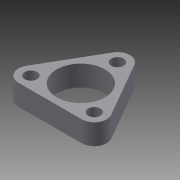
# Autodesk Inventor part: 零件3
Saved by Autodesk Inventor 2014 (Build 180170000, 170)
## iProperties
Created: 2018-10-26
Part Number: 零件3
Material: 常规
Document SubType Name: Modeling
Designer: Administrator
Density: 1 g/cm^3
Appearance: 默认
Author: Administrator
Autodesk Inventor part; units mm, degrees
ref_plane "YZ Plane" through (0, 0, 0) normal (1, 0, 0) x (0, 1, 0)
ref_plane "XZ Plane" through (0, 0, 0) normal (0, 1, 0) x (-1, 0, 0)
ref_plane "XY Plane" through (0, 0, 0) normal (0, 0, 1) x (1, 0, 0)
sketch "草图1" plane through (0, 0, 0) normal (0, 0, 1) x (1, 0, 0)
  line L0 (-7.7942, 31) -> (-30.7439, -8.75)
  line L1 (-22.9497, -22.25) -> (22.9497, -22.25)
  line L2 (7.7942, 31) -> (30.7439, -8.75)
  arc A0 (-30.7439, -8.75) -> (-22.9497, -22.25) centre (-22.9497, -13.25) ccw
  arc A1 (7.7942, 31) -> (-7.7942, 31) centre (0, 26.5) ccw
  arc A2 (22.9497, -22.25) -> (30.7439, -8.75) centre (22.9497, -13.25) ccw
  circle A3 centre (0, 0) radius 17.5
  circle A4 centre (0, 0) radius 26.5 construction
  circle A5 centre (-22.9497, -13.25) radius 4.5
  circle A6 centre (22.9497, -13.25) radius 4.5
  line L3 (0.1003, 40.3502) -> (0, 40.5239)
  line L4 (0, -39.0522) -> (0, 40.5239)
  line L5 (0, 0) -> (-22.9497, -13.25) construction
  line L6 (0, 0) -> (-28.9741, 0) construction
  circle A7 centre (0, 26.5) radius 4.5
  dimension "d0" = 9
  dimension "d1" = 9
  dimension "d2" = 9
  dimension "d3" = 53
  dimension "d4" = 35
  dimension "d5" = 30
  dimension "d6" = 9
  constraints: 14 end point, 8 centre point, 8 point on circle, 6 tangent, 5 coincident, 2 equal length, 2 perpendicular, 1 equal radius, 1 horizontal, 1 other
  measures "d0" radius of A0
  measures "d1" radius of A2
  measures "d2" diameter of A5
  measures "d3" diameter of A4
  measures "d4" diameter of A3
  measures "d5" angle of L5 L6
  measures "d6" diameter of A7
extrude "拉伸1" add sketch "草图1" along normal blind 15 contours A1 L4 A7 A3 L1 A0 L0 | A1 L2 A2 L1 L4 A3 A7
